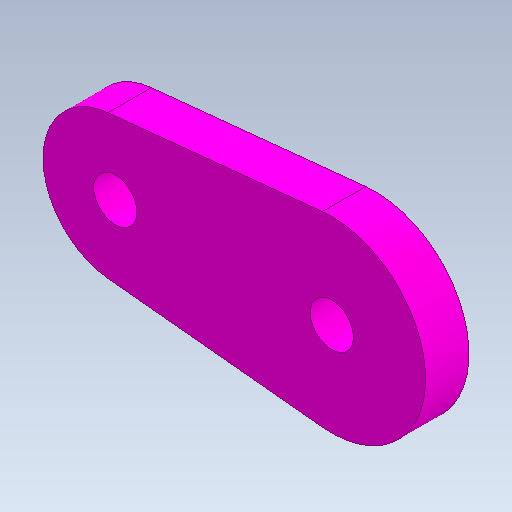
# Autodesk Inventor part: ウィング抑え
Saved by Autodesk Inventor 2020.2 (Build 242310000, 310)
## iProperties
Created: 2020-04-13
Part Number: ウィング抑え
Material: ポリカーボネート、スモーク
Document SubType Name: Modeling
Designer: aoyama
Density: 1.2 g/cm^3
Appearance: マゼンタ
Mass: 0.953504 g
Surface Area: 7.85108 cm^2
Volume: 0.794586 cm^3
Author: aoyama
Autodesk Inventor part; units mm, degrees
ref_plane "YZ Plane" through (0, 0, 0) normal (1, 0, 0) x (0, 1, 0)
ref_plane "XZ Plane" through (0, 0, 0) normal (0, 1, 0) x (-1, 0, 0)
ref_plane "XY Plane" through (0, 0, 0) normal (0, 0, 1) x (1, 0, 0)
sketch "スケッチ1" plane through (0, 0, 0) normal (0, 0, 1) x (1, 0, 0)
  line L0 (0, 0) -> (-15, 0) construction
  line L1 (0, 5) -> (-15, 5) construction
  line L2 (-15, -5) -> (0, -5) construction
  arc A0 (0, -5) -> (0, 5) centre (0, 0) ccw construction
  arc A1 (-15, 5) -> (-15, -5) centre (-15, 0) ccw
  circle A2 centre (-15, 0) radius 1.5
  circle A3 centre (0, 0) radius 1.5
  arc A4 (-0.65, 6.4674) -> (-0.65, -6.4674) centre (0, 0) ccw construction
  line L3 (-15.5, 4.9749) -> (-0.65, 6.4674)
  line L4 (-15.5, -4.9749) -> (-0.65, -6.4674)
  arc A5 (-0.65, -6.4674) -> (-0.65, 6.4674) centre (0, 0) ccw
  point P0 (-7.5, 0)
  dimension "d0" = 15
  dimension "d1" = 10
  dimension "d2" = 3
  dimension "d3" = 3
  dimension "d4" = 13
  constraints: 12 end point, 9 point on circle, 6 centre point, 6 tangent, 3 coincident, 2 symmetric about line, 1 horizontal, 1 midpoint, 1 parallel
  measures "d0" distance of L0.start L0.end
  measures "d1" diameter of A1
  measures "d2" diameter of A2
  measures "d3" diameter of A3
  measures "d4" diameter of A4
extrude "押し出し1" add sketch "スケッチ1" along normal blind 3
